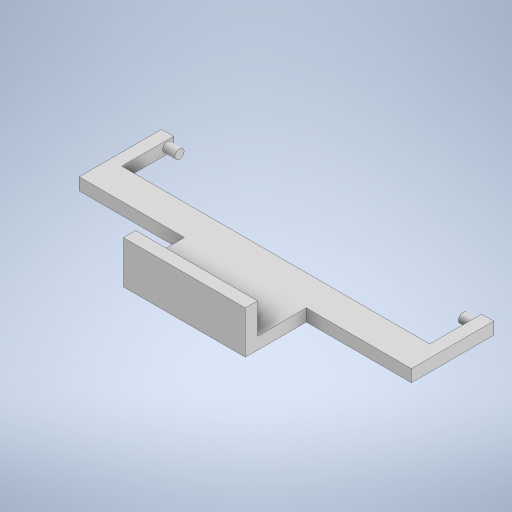
# Autodesk Inventor part: крюк
Saved by Autodesk Inventor 2023.2 (Build 272271000, 271)
## iProperties
Created: 2024-01-18
Part Number: крюк
Material: Типовые
Document SubType Name: Modeling
Designer: парпа
Density: 1 g/cm^3
Appearance: По умолчанию
Author: парпа
Autodesk Inventor part; units mm, degrees
ref_plane "YZ Plane" through (0, 0, 0) normal (1, 0, 0) x (0, 1, 0)
ref_plane "XZ Plane" through (0, 0, 0) normal (0, 1, 0) x (-1, 0, 0)
ref_plane "XY Plane" through (0, 0, 0) normal (0, 0, 1) x (1, 0, 0)
sketch "Эскиз1" plane through (0, 0, 0) normal (0, 1, 0) x (-1, 0, 0)
  line L0 (0, 0) -> (47.5295, 0)
  line L1 (0, 0) -> (-53.4705, 0)
  line L2 (47.5295, 0) -> (-53.4705, 0)
  line L3 (-53.4705, 0) -> (-53.4705, 10)
  line L4 (-53.4705, 10) -> (47.5295, 10)
  line L5 (47.5295, 10) -> (47.5295, 0)
  dimension "d0" = 101
  dimension "d1" = 10
  constraints: 12 end point, 3 horizontal, 2 parallel, 1 perpendicular
  measures "d0" distance of L0.end L1.end
  measures "d1" distance of L4.end L0.end
extrude "Выдавливание1" add sketch "Эскиз1" along normal blind 4
sketch "Эскиз2" plane through (-47.5295, 0, 10) normal (0, 0, 1) x (1, 0, 0)
  line L0 (0, 4) -> (101, 4) projected
  line L1 (0, 4) -> (50.5, 4)
  line L2 (30.5, 0) -> (70.5, 0)
  line L3 (70.5, 0) -> (70.5, 4)
  line L4 (70.5, 4) -> (30.5, 4)
  line L5 (30.5, 4) -> (30.5, 0)
  line L6 (30.5, 0) -> (70.5, 4) construction
  line L7 (70.5, 0) -> (30.5, 4) construction
  point P0 (47.5295, 0)
  point P1 (50.5, 2)
  point P2 (30.5, 2)
  point P3 (70.5, 2)
  dimension "d4" = 50.5
  dimension "d5" = 40
  dimension "d6" = 4
  constraints: 14 end point, 6 midpoint, 2 parallel, 1 horizontal, 1 perpendicular, 1 point on line
  measures "d4" distance of L0.start point (50.5, 4)
  measures "d5" distance of point (30.5, 2) point (70.5, 2)
  measures "d6" distance of L2.end L3.end
extrude "Выдавливание2" add sketch "Эскиз2" along normal blind 20
sketch "Эскиз3" plane through (0, 4, 0) normal (0, 1, 0) x (1, 0, 0)
  line L0 (-17.0295, -30) -> (22.9705, -30) projected
  line L1 (22.9705, -10) -> (22.9705, -30) projected
  line L2 (-17.0295, -30) -> (22.9705, -30)
  line L3 (22.9705, -30) -> (22.9705, -26)
  line L4 (22.9705, -26) -> (-17.0295, -26)
  line L5 (-17.0295, -26) -> (-17.0295, -30)
  point P0 (0, 0)
  dimension "d9" = 4
  constraints: 8 end point, 2 parallel, 1 horizontal, 1 perpendicular, 1 point on line
  measures "d9" distance of L4.end L0.start
extrude "Выдавливание3" add sketch "Эскиз3" along normal blind 10
sketch "Эскиз4" plane through (53.4705, 0, 10) normal (1, 0, 0) x (0, 0, -1)
  line L0 (0, 4) -> (10, 4) projected
  line L1 (0, 4) -> (27, 4)
  line L2 (27, 4) -> (27, 0)
  line L3 (27, 0) -> (0, 0)
  line L4 (0, 0) -> (0, 4)
  line L5 (10, 0) -> (10, 4) projected
  dimension "d12" = 17
  constraints: 8 end point, 2 parallel, 1 horizontal, 1 perpendicular
  measures "d12" distance between parallel lines of L2 L5
extrude "Выдавливание4" add sketch "Эскиз4" along normal blind 4
sketch "Эскиз5" plane through (-47.5295, 0, 0) normal (-1, 0, 0) x (0, 0, 1)
  line L0 (-17, 4) -> (0, 4) projected
  line L1 (10, 0) -> (-17, 0)
  line L2 (-17, 0) -> (-17, 4)
  line L3 (-17, 4) -> (10, 4)
  line L4 (10, 4) -> (10, 0)
  point P0 (0, 0)
  point P1 (0, 4)
  constraints: 8 end point, 2 parallel, 1 horizontal, 1 perpendicular
extrude "Выдавливание5" add sketch "Эскиз5" along normal blind 4
sketch "Эскиз6" plane through (-47.5295, 0, 0) normal (1, 0, 0) x (0, 0, -1)
  circle A0 centre (14.9, 2.0073) radius 1.5
  line L0 (14.9, 2.0073) -> (17, 2)
  line L1 (17, 4) -> (17, 0) projected
  point P0 (0, 0)
  dimension "d17" = 3
  dimension "d18" = 2.1
  constraints: 2 end point, 1 centre point, 1 midpoint
  measures "d17" diameter of A0
  measures "d18" distance of L0.start L0.end
extrude "Выдавливание6" add sketch "Эскиз6" along normal blind 4
sketch "Эскиз7" plane through (53.4705, 0, 10) normal (-1, 0, 0) x (0, 0, 1)
  circle A0 centre (-24.9, 2.0073) radius 1.5 projected
  circle A1 centre (-24.9, 2.0073) radius 1.5
  point P0 (-10, 0)
  constraints: 1 centre point, 1 coincident
extrude "Выдавливание7" add sketch "Эскиз7" along normal blind 4
